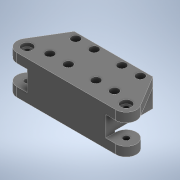
# Autodesk Inventor part: YAxisEndBlock_10mm
Saved by Autodesk Inventor 2022 (Build 260153000, 153)
## iProperties
Created: 2021-06-16
Part Number: YAxisEndBlock_10mm
Material: Generic
Document SubType Name: Modeling
Designer: burgessb
Density: 1 g/cm^3
Appearance: Gray
Author: burgessb
Autodesk Inventor part; units mm, degrees
ref_plane "YZ Plane" through (0, 0, 0) normal (1, 0, 0) x (0, 1, 0)
ref_plane "XZ Plane" through (0, 0, 0) normal (0, 1, 0) x (-1, 0, 0)
sketch "Sketch1" plane through (0, 0, 0) normal (0, 1, 0) x (-1, 0, 0)
  line L0 (0, 0) -> (35, 0)
  line L1 (35, 0) -> (35, 40)
  line L2 (35, 40) -> (0, 40)
  line L3 (0, 40) -> (0, 0)
  line L4 (50, 0) -> (85, 0)
  line L5 (85, 0) -> (85, 40)
  line L6 (85, 40) -> (50, 40)
  line L7 (50, 40) -> (50, 0)
  line L8 (50, 40) -> (35, 40)
  line L9 (50, 0) -> (35, 0)
  line L10 (0, 40) -> (0, 51)
  line L11 (0, 51) -> (85, 51)
  line L12 (85, 51) -> (85, 40)
  dimension "d0" = 40
  dimension "d1" = 35
  dimension "d2" = 40
  dimension "d3" = 35
  dimension "d4" = 50
  dimension "d5" = 0
  dimension "d6" = 11
  constraints: 26 end point, 4 parallel, 4 perpendicular, 2 horizontal, 1 vertical
  measures "d0" distance of L2.end L0.start
  measures "d1" distance of L0.start L0.end
  measures "d2" distance of L6.end L4.start
  measures "d3" distance of L4.start L4.end
  measures "d4" distance between parallel lines of L3 L7
  measures "d5" distance between parallel lines of L0 L4
  measures "d6" distance of L2.end L10.end
extrude "Extrusion1" add sketch "Sketch1" along normal blind 30
sketch "Sketch2" plane through (0, 0, 0) normal (0, -1, 0) x (1, 0, 0)
  line L0 (-85, 0) -> (-85, 51) projected
  line L1 (0, 0) -> (-85, 0) projected
  line L2 (0, 51) -> (0, 0) projected
  line L3 (-85, 51) -> (0, 51) projected
  line L4 (-85, 51) -> (0, 51) projected
  line L5 (-85, 0) -> (-85, 51) projected
  line L6 (0, 51) -> (-85, 51)
  line L7 (-85, 51) -> (-85, 41)
  line L8 (-85, 41) -> (0, 41)
  line L9 (0, 41) -> (0, 51)
  dimension "d9" = 10
  constraints: 8 end point, 2 parallel, 1 horizontal, 1 perpendicular, 1 point on line
  measures "d9" distance of L7.end L6.end
extrude "Extrusion2" add sketch "Sketch2" along normal blind 12 contours L0 L3 L2 L8
sketch "Sketch3" plane through (0, 0, 0) normal (0, 0, -1) x (-1, 0, 0)
  line L0 (0, 0) -> (85, 0) projected
  line L1 (85, 0) -> (85, 30) projected
  line L2 (0, 30) -> (85, 30) projected
  line L3 (0, 0) -> (0, 30) projected
  circle A0 centre (17.5, 10) radius 5.25
  circle A1 centre (67.5, 10) radius 5.25
  dimension "d12" = 10.5
  dimension "d13" = 10.5
  dimension "d14" = 10
  dimension "d15" = 10
  dimension "d16" = 50
  dimension "d17" = 17.5
  dimension "d18" = 17.5
  constraints: 2 centre point
  measures "d12" diameter of A0
  measures "d13" diameter of A1
  measures "d14" distance from line of L0 A0.centre
  measures "d15" distance from line of L0 A1.centre
  measures "d16" distance of A0.centre A1.centre
  measures "d17" distance from line of L3 A0.centre
  measures "d18" distance from line of L1 A1.centre
extrude "Extrusion3" cut sketch "Sketch3" against normal blind 30 contours A0 | A1
sketch "Sketch4" plane through (0, 30, 0) normal (0, 1, 0) x (1, 0, 0)
  line L0 (-85, 0) -> (-85, -51) projected
  line L1 (-85, -51) -> (0, -51) projected
  line L2 (0, -51) -> (0, 0) projected
  line L3 (0, 0) -> (-85, 0) projected
  line L4 (0, -51) -> (-85, -51) projected
  line L5 (-42.5, -51) -> (-42.5, 0) construction
  line L6 (0, 0) -> (-85, 0) projected
  circle A0 centre (11.1, -39.9) radius 3.25
  circle A1 centre (25, -51) radius 6.1 construction
  circle A2 centre (11.1, -39.9) radius 5
  circle A3 centre (11.1, -39.9) radius 11.1
  line L7 (0, -51) -> (11.1, -51)
  line L8 (0, -41) -> (-85, -41) projected
  line L9 (0, -41) -> (0, 0) projected
  line L10 (0, 0) -> (20.6053, -34.1677)
  circle A4 centre (-96.1, -39.9) radius 3.25
  circle A5 centre (-110, -51) radius 6.1 construction
  circle A6 centre (-96.1, -39.9) radius 5
  circle A7 centre (-96.1, -39.9) radius 11.1
  line L11 (-85, -51) -> (-96.1, -51)
  line L12 (-85, 0) -> (-105.6053, -34.1677)
  dimension "d22" = 6.5
  dimension "d23" = 11.1
  dimension "d24" = 12.2
  dimension "d25" = 25
  dimension "d26" = 0
  dimension "d27" = 10
  dimension "d28" = 11.1
  dimension "d30" = 22.2
  constraints: 10 end point, 8 centre point, 7 symmetric about line, 4 coincident, 4 point on circle, 2 midpoint, 2 tangent, 4 other
  measures "d22" diameter of A0
  measures "d23" distance from line of L2 A0.centre
  measures "d24" diameter of A1
  measures "d25" distance of L1.end A1.centre
  measures "d26" vertical distance of L1.end A1.centre
  measures "d27" diameter of A2
  measures "d28" vertical distance of A1.centre A0.centre
  measures "d30" diameter of A3
extrude "Extrusion4" add sketch "Sketch4" against normal blind 10 contours L0 A7 L12 | A7 | L0 L11 A7 | L10 A3 L2 | A3 L7 L2 | A3 | A2 | A6
ref_plane "Work Plane1" through (0, -12, 0) normal (0, 1, 0) x (1, 0, 0)
sketch "Sketch5" plane through (0, -12, 0) normal (0, 1, 0) x (1, 0, 0)
  arc A0 (11.1, -51) -> (20.6053, -34.1677) centre (11.1, -39.9) ccw projected
  circle A1 centre (11.1, -39.9) radius 3.25 projected
  line L0 (0, -41) -> (0, -51) projected
  line L1 (0, -41) -> (0, 0) projected
  circle A2 centre (11.1, -39.9) radius 3.25 projected
  circle A3 centre (11.1, -39.9) radius 11.1
  line L2 (11.1, -51) -> (0, -51) projected
  line L3 (-85, -41) -> (0, -41) projected
  arc A4 (-105.6053, -34.1677) -> (-96.1, -51) centre (-96.1, -39.9) ccw projected
  circle A5 centre (-96.1, -39.9) radius 3.25 projected
  line L4 (-85, -51) -> (-96.1, -51) projected
  line L5 (-85, -51) -> (-85, -41) projected
  line L6 (-85, 0) -> (-85, -41) projected
  circle A6 centre (-96.1, -39.9) radius 11.1
  point P0 (20.6053, -34.1677)
  point P1 (0, -39.9)
  point P2 (-85, -39.9)
  point P3 (-105.6053, -34.1677)
  constraints: 2 centre point, 2 coincident, 2 concentric
extrude "Extrusion5" add sketch "Sketch5" along normal blind 10
sketch "Sketch6" plane through (0, 30, 0) normal (0, 1, 0) x (1, 0, 0)
  circle A0 centre (-96.1, -39.9) radius 3.25 projected
  circle A1 centre (11.1, -39.9) radius 3.25 projected
  circle A2 centre (11.1, -39.9) radius 5.75
  circle A3 centre (-96.1, -39.9) radius 5.75
  point P0 (0, 0)
  dimension "d36" = 11.5
  dimension "d37" = 11.5
  constraints: 2 centre point, 2 coincident
  measures "d36" diameter of A2
  measures "d37" diameter of A3
extrude "Extrusion6" cut sketch "Sketch6" against normal blind 4
sketch "Sketch7" plane through (0, -12, 0) normal (0, -1, 0) x (1, 0, 0)
  circle A0 centre (11.1, 39.9) radius 3.25 projected
  circle A1 centre (-96.1, 39.9) radius 3.25 projected
  circle A2 centre (11.1, 39.9) radius 5.75 projected
  circle A3 centre (11.1, 39.9) radius 5.75 projected
  circle A4 centre (-96.1, 39.9) radius 5.75 projected
  point P0 (0, 0)
extrude "Extrusion7" cut sketch "Sketch7" against normal blind 4
sketch "Sketch8" plane through (0, 0, 0) normal (0, -1, 0) x (1, 0, 0)
  line L0 (0, 41) -> (-85, 41) projected
  line L1 (-85, 0) -> (-85, 41) projected
  line L2 (0, 0) -> (-85, 0) projected
  line L3 (0, 41) -> (0, 0) projected
  circle A0 centre (-7.5, 6) radius 2.25
  circle A1 centre (-27.5, 6) radius 2.25
  circle A2 centre (-7.5, 34) radius 2.25
  circle A3 centre (-27.5, 34) radius 2.25
  line L4 (0, 0) -> (-85, 0) projected
  line L5 (-42.5, 0) -> (-42.5, 41) construction
  line L6 (-85, 41) -> (0, 41) projected
  circle A4 centre (-77.5, 6) radius 2.25
  circle A5 centre (-57.5, 6) radius 2.25
  circle A6 centre (-77.5, 34) radius 2.25
  circle A7 centre (-57.5, 34) radius 2.25
  dimension "d42" = 4.5
  dimension "d45" = 20
  dimension "d48" = 28
  dimension "d51" = 6
  dimension "d52" = 7.5
  constraints: 8 centre point, 4 symmetric about line, 2 end point, 2 midpoint, 1 horizontal, 1 vertical, 10 other
  measures "d42" diameter of A0
  measures "d45" distance of A0.centre A1.centre
  measures "d48" distance of A0.centre A2.centre
  measures "d51" distance from line of L2 A0.centre
  measures "d52" distance from line of L3 A0.centre
extrude "Extrusion8" cut sketch "Sketch8" against normal through all contours A0 | A1 | A2 | A3 | A4 | A5 | A6 | A7
sketch "Sketch9" plane through (0, 30, 0) normal (0, 1, 0) x (1, 0, 0)
  line L0 (-12.25, 0) -> (-12.25, -30) projected
  circle A0 centre (-7.5, -34) radius 2.25 projected
  circle A1 centre (-77.5, -6) radius 2.25 projected
  circle A2 centre (-57.5, -6) radius 2.25 projected
  circle A3 centre (-7.5, -6) radius 2.25 projected
  circle A4 centre (-27.5, -34) radius 2.25 projected
  circle A5 centre (-77.5, -34) radius 2.25 projected
  circle A6 centre (-57.5, -34) radius 2.25 projected
  circle A7 centre (-27.5, -6) radius 2.25 projected
  circle A8 centre (-96.1, -39.9) radius 5.75 projected
  circle A9 centre (11.1, -39.9) radius 5.75 projected
  line L1 (-96.1, -51) -> (11.1, -51) projected
  arc A10 (11.1, -51) -> (20.6053, -34.1677) centre (11.1, -39.9) ccw projected
  line L2 (20.6053, -34.1677) -> (0, 0) projected
  line L3 (0, 0) -> (-85, 0) projected
  line L4 (-85, 0) -> (-105.6053, -34.1677) projected
  arc A11 (-105.6053, -34.1677) -> (-96.1, -51) centre (-96.1, -39.9) ccw projected
  circle A12 centre (-7.5, -6) radius 4.5
  circle A13 centre (-7.5, -34) radius 4.5
  circle A14 centre (-27.5, -34) radius 2.25 projected
  circle A15 centre (-27.5, -34) radius 4.5
  circle A16 centre (-27.5, -6) radius 2.25 projected
  circle A17 centre (-27.5, -6) radius 4.5
  circle A18 centre (-57.5, -6) radius 2.25 projected
  circle A19 centre (-57.5, -6) radius 4.5
  circle A20 centre (-57.5, -34) radius 4.5
  circle A21 centre (-77.5, -34) radius 2.25 projected
  circle A22 centre (-77.5, -34) radius 4.5
  circle A23 centre (-77.5, -6) radius 2.25 projected
  circle A24 centre (-77.5, -6) radius 4.5
  dimension "d55" = 9
  dimension "d56" = 9
  dimension "d57" = 9
  dimension "d58" = 9
  dimension "d59" = 9
  dimension "d60" = 9
  dimension "d61" = 9
  dimension "d62" = 9
  constraints: 8 centre point, 8 coincident
  measures "d55" diameter of A12
  measures "d56" diameter of A13
  measures "d57" diameter of A15
  measures "d58" diameter of A17
  measures "d59" diameter of A19
  measures "d60" diameter of A20
  measures "d61" diameter of A22
  measures "d62" diameter of A24
extrude "Extrusion9" cut sketch "Sketch9" against normal blind 20 contours A0 | A1 | A2 | A3 | A4 | A5 | A6 | A7 | A12 | A13 | A15 | A17 | A19 | A20 | A22 | A24
equation "\"d17\" = d18"
equation "\"d23\" = 0.5 * d30"
equation "\"d28\" = 0.5 * d27 + 0.5 * d24"
equation "\"d30\" = 2 * d28"
equation "\"d31\" = d27"
equation "\"d56\" = d55"
equation "\"d57\" = d55"
equation "\"d58\" = d55"
equation "\"d59\" = d55"
equation "\"d60\" = d55"
equation "\"d61\" = d55"
equation "\"d62\" = d55"
body "Solid1"
